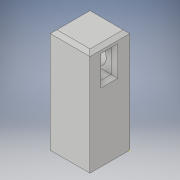
# Autodesk Inventor part: XTower
Saved by Autodesk Inventor 2018 (Build 220112000, 112)
## iProperties
Created: 2020-03-14
Part Number: XTower
Material: Generic
Document SubType Name: Modeling
Designer: natha
Density: 1 g/cm^3
Appearance: Default
Author: natha
Autodesk Inventor part; units mm, degrees
ref_plane "YZ Plane" through (0, 0, 0) normal (1, 0, 0) x (0, 1, 0)
ref_plane "XZ Plane" through (0, 0, 0) normal (0, 1, 0) x (-1, 0, 0)
ref_plane "XY Plane" through (0, 0, 0) normal (0, 0, 1) x (1, 0, 0)
sketch "Sketch1" plane through (0, 0, 0) normal (0, 1, 0) x (-1, 0, 0)
  line L0 (0, 0) -> (38.1, 0)
  line L1 (38.1, 0) -> (38.1, -38.1)
  line L2 (38.1, -38.1) -> (0, -38.1)
  line L3 (0, -38.1) -> (0, 0)
  dimension "d0" = 38.1
  dimension "d1" = 38.1
  constraints: 8 end point, 2 parallel, 1 horizontal, 1 perpendicular
  measures "d0" distance of L1.end L2.end
  measures "d1" distance of L0.end L1.end
extrude "Extrusion1" add sketch "Sketch1" along normal blind 100
sketch "Sketch2" plane through (0, 0, -38.1) normal (0, 0, -1) x (-1, 0, 0)
  circle A0 centre (19.05, 80) radius 11.15
  line L0 (0, 100) -> (38.1, 100) projected
  line L1 (0, 0) -> (0, 100) projected
  dimension "d4" = 22.3
  dimension "d5" = 20
  dimension "d6" = 19.05
  constraints: 1 centre point
  measures "d4" diameter of A0
  measures "d5" distance from line of L0 A0.centre
  measures "d6" distance from line of L1 A0.centre
sketch "Sketch3" plane through (0, 0, -38.1) normal (0, 0, -1) x (-1, 0, 0)
  point P0 (0, 0)
extrude "Extrusion2" cut sketch "Sketch2" against normal blind 33.02
sketch "Sketch4" plane through (0, 0, 0) normal (1, 0, 0) x (0, 0, -1)
  line L0 (13.4535, 68.7) -> (23.4535, 68.7)
  line L1 (23.4535, 68.7) -> (23.4535, 91)
  line L2 (23.4535, 91) -> (13.4535, 91)
  line L3 (13.4535, 91) -> (13.4535, 68.7)
  line L4 (13.4535, 68.7) -> (23.4535, 91) construction
  line L5 (23.4535, 68.7) -> (13.4535, 91) construction
  line L6 (0, 100) -> (38.1, 100) projected
  point P0 (0, 0)
  point P1 (18.4535, 79.85)
  dimension "d9" = 10
  dimension "d10" = 22.3
  dimension "d11" = 9
  constraints: 12 end point, 2 midpoint, 2 parallel, 1 horizontal, 1 perpendicular
  measures "d9" distance of L2.end L1.end
  measures "d10" distance of L1.end L0.end
  measures "d11" distance between parallel lines of L6 L2
extrude "Extrusion3" cut sketch "Sketch4" against normal blind 19.05
chamfer "Chamfer1" distance 3.175 angle 45 8 edges at (0, 91, -18.4535) (0, 68.7, -18.4535) (0, 79.85, -13.4535) (0, 79.85, -23.4535) (0, 100, -19.05) (-19.05, 100, -38.1) (-38.1, 100, -19.05) (-19.05, 100, 0)
body "Solid1"
